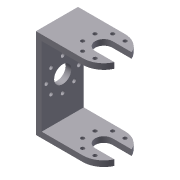
# Autodesk Inventor part: Shoulder
Saved by Autodesk Inventor 2011 (Build 150239000, 239)
## iProperties
Created: 2010-11-22
Part Number: Shoulder
Document SubType Name: Modeling
Designer: Milton
Density: 2.71 g/cm^3
Mass: 16.079 g
Surface Area: 53.1427 cm^2
Volume: 5.93321 cm^3
Material: Aluminum-6061
Author: Milton
Autodesk Inventor part; units mm, degrees
ref_plane "YZ Plane" through (0, 0, 0) normal (1, 0, 0) x (0, 1, 0)
ref_plane "XZ Plane" through (0, 0, 0) normal (0, 1, 0) x (-1, 0, 0)
ref_plane "XY Plane" through (0, 0, 0) normal (0, 0, 1) x (1, 0, 0)
sketch "Sketch1" plane through (0, 0, 0) normal (0, 0, 1) x (1, 0, 0)
  line L0 (5.3975, 5.374) -> (29.8975, 5.374)
  line L1 (5.3975, 27.374) -> (29.8975, 27.374)
  line L2 (5.3975, 5.374) -> (5.3975, 27.374)
  arc A0 (29.8975, 20.874) -> (29.8975, 11.874) centre (29.8975, 16.374) ccw
  line L3 (29.8975, 20.874) -> (39.9349, 20.874)
  line L4 (29.8975, 11.874) -> (39.9349, 11.874)
  arc A1 (29.8975, 5.374) -> (39.9349, 11.874) centre (29.8975, 16.374) ccw
  arc A2 (39.9349, 20.874) -> (29.8975, 27.374) centre (29.8975, 16.374) ccw
  point P0 (0, 0)
  dimension "d0" = 9
  constraints: 10 end point, 6 point on circle, 3 centre point, 2 perpendicular, 2 tangent, 1 coincident, 1 parallel
  measures "d0" diameter of A0
extrude "Extrusion1" add sketch "Sketch1" along normal blind 47
sketch "Sketch2" plane through (5.3975, 5.374, 0) normal (0, -1, 0) x (1, 0, 0)
  line L0 (24.5, 47) -> (0, 47) projected
  line L1 (0, 0) -> (0, 47) projected
  line L2 (24.5, 0) -> (24.5, 47) projected
  line L3 (3, 44) -> (34.5374, 44)
  line L4 (34.5374, 0) -> (34.5374, 47) projected
  line L5 (34.5374, 44) -> (34.5374, 3)
  line L6 (3, 44) -> (3, 3)
  line L7 (3, 3) -> (34.5374, 3)
  line L8 (34.5374, 0) -> (24.5, 0) projected
  point P0 (-5.3975, 0)
  dimension "d3" = 3
  dimension "d4" = 3
  dimension "d5" = 3
  constraints: 8 end point, 2 perpendicular, 2 point on line, 1 parallel
  measures "d3" distance between parallel lines of L1 L6
  measures "d4" distance between parallel lines of L0 L3
  measures "d5" distance between parallel lines of L8 L7
extrude "Extrusion2" cut sketch "Sketch2" against normal through all contours L7 L6 L3 L2 | L2 L3 L4 L7
sketch "Sketch3" plane through (5.3975, 5.374, 0) normal (-1, 0, 0) x (0, 0, 1)
  circle A0 centre (23.5, 11) radius 4.5
  point P0 (0, -5.374)
  dimension "d8" = 9
  constraints: 1 centre point
  measures "d8" diameter of A0
extrude "Extrusion3" cut sketch "Sketch3" against normal through all
sketch "Sketch4" plane through (0, 0, 0) normal (0, 0, -1) x (-1, 0, 0)
  line L0 (-5.3975, 5.374) -> (-29.8975, 5.374) projected
  arc A0 (-29.8975, 27.374) -> (-39.9349, 20.874) centre (-29.8975, 16.374) ccw projected
  arc A1 (-29.8975, 11.874) -> (-29.8975, 20.874) centre (-29.8975, 16.374) ccw projected
  arc A2 (-39.9349, 11.874) -> (-29.8975, 5.374) centre (-29.8975, 16.374) ccw projected
  circle A3 centre (-22.0445, 19.6268) radius 1
  line L1 (-29.8975, 16.374) -> (-22.0445, 19.6268)
  circle A4 centre (-26.6447, 24.2269) radius 1
  circle A5 centre (-33.1503, 24.2269) radius 1
  circle A6 centre (-37.7505, 19.6268) radius 1
  circle A7 centre (-37.7505, 13.1211) radius 1
  circle A8 centre (-33.1503, 8.521) radius 1
  circle A9 centre (-26.6447, 8.521) radius 1
  circle A10 centre (-22.0445, 13.1211) radius 1
  point P0 (0, 0)
  dimension "d11" = 2
  dimension "d12" = 8.5
  dimension "d13" = 22.5
  dimension "d16" = 360
  constraints: 8 centre point, 2 end point, 17 other
  measures "d11" diameter of A3
  measures "d12" distance of L1.end A0.centre
  measures "d13" angle of L0 L1
extrude "Extrusion4" cut sketch "Sketch4" against normal through all contours A3 | A4 | A5 | A8 | A9 | A10
sketch "Sketch5" plane through (8.3975, 5.374, 44) normal (1, 0, 0) x (0, 0, -1)
  circle A0 centre (20.5, 11) radius 4.5 projected
  circle A1 centre (20.5, 19.5) radius 1
  point P0 (44, -5.374)
  dimension "d20" = 2
  dimension "d21" = 8.5
  constraints: 1 centre point
  measures "d20" diameter of A1
  measures "d21" distance of A1.centre A0.centre
extrude "Extrusion5" cut sketch "Sketch5" against normal through all contours A1
pattern_circular "Circular Pattern1" count 8 over 360 about axis through (5.3975, 16.374, 23.5) along (1, 0, 0) of "Extrusion5"
body "Solid1"
